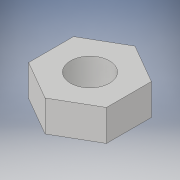
# Autodesk Inventor part: Bag motor nut
Saved by Autodesk Inventor 2017 (Build 210142000, 142)
## iProperties
Created: 2016-09-26
Part Number: Bag motor nut
Material: Generic
Document SubType Name: Modeling
Designer: hanso
Density: 1 g/cm^3
Appearance: Default
Author: hanso
Autodesk Inventor part; units mm, degrees
ref_plane "YZ Plane" through (0, 0, 0) normal (1, 0, 0) x (0, 1, 0)
ref_plane "XZ Plane" through (0, 0, 0) normal (0, 1, 0) x (-1, 0, 0)
ref_plane "XY Plane" through (0, 0, 0) normal (0, 0, 1) x (1, 0, 0)
sketch "Sketch1" plane through (0, 0, 0) normal (0, 1, 0) x (-1, 0, 0)
  line L0 (0, -4.5827) -> (-3.9687, -2.2914)
  line L1 (-3.9687, -2.2914) -> (-3.9688, 2.2914)
  line L2 (-3.9688, 2.2914) -> (0, 4.5827)
  line L3 (0, 4.5827) -> (3.9687, 2.2914)
  line L4 (3.9687, 2.2914) -> (3.9688, -2.2914)
  line L5 (3.9688, -2.2914) -> (0, -4.5827)
  point P0 (0, 0)
  point P1 (0, 0)
  dimension "d0" = 3.9688
  constraints: 12 end point, 1 coincident, 13 other
  measures "d0" distance from line of point (0, 0) L4
extrude "Extrusion1" add sketch "Sketch1" along normal blind 3.175
sketch "Sketch2" plane through (0, 3.175, 0) normal (0, 1, 0) x (1, 0, 0)
  point P0 (0, 0)
  point P1 (0, 0)
  constraints: 1 coincident
hole "Hole1" at (0, 3.175, 0) direction (0, -1, 0) diameter 3.9688 end through all
body "Solid1"
